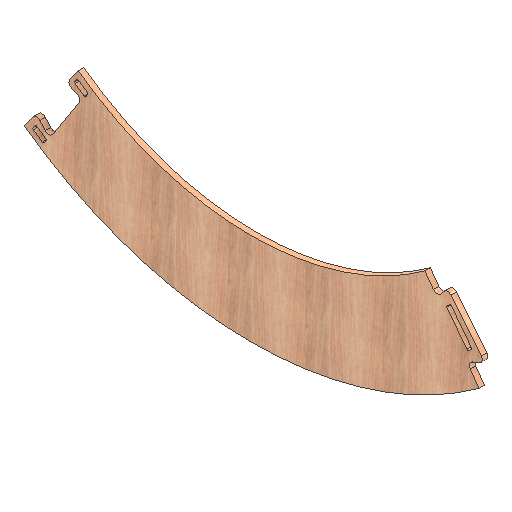
# Autodesk Inventor part: Platform D3
Saved by Autodesk Inventor 2021 (Build 250183000, 183)
## iProperties
Created: 2020-05-09
Part Number: Platform D3
Material: Wood (Birch)
Document SubType Name: Modeling
Designer: Dan Wikman
Density: 0.55 g/cm^3
Appearance: Birch - Natural Polished
Mass: 4202.36 g
Surface Area: 9235.8 cm^2
Volume: 7640.65 cm^3
Autodesk Inventor part; units mm, degrees
ref_plane "YZ Plane" through (0, 0, 0) normal (1, 0, 0) x (0, 1, 0)
ref_plane "XZ Plane" through (0, 0, 0) normal (0, 1, 0) x (-1, 0, 0)
ref_plane "XY Plane" through (0, 0, 0) normal (0, 0, 1) x (1, 0, 0)
sketch "CONTOURS" plane through (0, 0, 0) normal (0, 0, 1) x (1, 0, 0)
  line L0 (1512.926, 262.3244) -> (1483.7011, 302.5491)
  arc A0 (1490.3116, 325.9808) -> (1483.7011, 302.5491) centre (1496.2408, 311.6597) ccw
  line L1 (1490.3116, 325.9808) -> (1515.055, 336.2252)
  arc A1 (1515.055, 336.2252) -> (1520.7765, 358.748) centre (1509.5083, 349.6224) ccw
  line L2 (1520.7765, 358.748) -> (1420.6454, 482.3882)
  arc A2 (1420.6454, 482.3882) -> (1397.875, 482.0914) centre (1409.3772, 473.2625) ccw
  line L3 (1397.875, 482.0914) -> (1387.5892, 468.6913)
  arc A3 (1362.754, 469.0184) -> (1387.5892, 468.6913) centre (1375.2938, 478.1291) ccw
  line L4 (1362.754, 469.0184) -> (1334.3843, 508.066)
  arc A4 (193.4245, 508.066) -> (1334.3843, 508.066) centre (763.9044, 1294.3771) ccw
  line L5 (193.4245, 508.066) -> (165.0547, 469.0184)
  arc A5 (165.0547, 469.0184) -> (171.943, 446.828) centre (176.7854, 460.4955) ccw
  line L6 (171.943, 446.828) -> (187.8658, 441.1866)
  arc A6 (195.6892, 418.1351) -> (187.8658, 441.1866) centre (182.6894, 426.5765) ccw
  line L7 (195.6892, 418.1351) -> (109.0426, 284.6979)
  arc A7 (84.2549, 283.0747) -> (109.0426, 284.6979) centre (96.0429, 293.1392) ccw
  line L8 (84.2549, 283.0747) -> (66.8658, 303.4414)
  arc A8 (66.8658, 303.4414) -> (44.1076, 302.5491) centre (55.8384, 294.0262) ccw
  line L9 (44.1076, 302.5491) -> (14.8827, 262.3244)
  arc A9 (14.8827, 262.3244) -> (1512.926, 262.3244) centre (763.9044, 1294.1149) ccw
  constraints: 20 end point, 20 point on circle, 10 centre point
sketch "HOLES" plane through (0, 0, 0) normal (0, 0, 1) x (1, 0, 0)
  line L0 (224.6944, 455.9957) -> (218.4625, 446.9313)
  arc A0 (212.9002, 445.9014) -> (218.4625, 446.9313) centre (215.1664, 449.1975) ccw
  line L1 (212.9002, 445.9014) -> (183.2349, 466.2968)
  arc A1 (182.205, 471.8591) -> (183.2349, 466.2968) centre (185.5011, 469.5929) ccw
  line L2 (182.205, 471.8591) -> (188.4369, 480.9234)
  arc A2 (193.9992, 481.9534) -> (188.4369, 480.9234) centre (191.733, 478.6573) ccw
  line L3 (193.9992, 481.9534) -> (223.6644, 461.558)
  arc A3 (224.6944, 455.9957) -> (223.6644, 461.558) centre (221.3983, 458.2619) ccw
  line L4 (87.0245, 255.754) -> (80.7926, 246.6896)
  arc A4 (75.2303, 245.6596) -> (80.7926, 246.6896) centre (77.4965, 248.9557) ccw
  line L5 (75.2303, 245.6596) -> (45.5651, 266.055)
  arc A5 (44.5351, 271.6173) -> (45.5651, 266.055) centre (47.8312, 269.3511) ccw
  line L6 (44.5351, 271.6173) -> (50.767, 280.6817)
  arc A6 (56.3293, 281.7117) -> (50.767, 280.6817) centre (54.0631, 278.4155) ccw
  line L7 (56.3293, 281.7117) -> (85.9946, 261.3163)
  arc A7 (87.0245, 255.754) -> (85.9946, 261.3163) centre (83.7284, 258.0201) ccw
  line L8 (1487.4439, 359.9016) -> (1478.716, 353.2066)
  arc A8 (1473.1076, 353.9459) -> (1478.716, 353.2066) centre (1476.2814, 356.3804) ccw
  line L9 (1473.1076, 353.9459) -> (1406.7666, 440.4321)
  arc A9 (1407.5058, 446.0405) -> (1406.7666, 440.4321) centre (1409.9404, 442.8667) ccw
  line L10 (1407.5058, 446.0405) -> (1416.2338, 452.7354)
  arc A10 (1421.8421, 451.9962) -> (1416.2338, 452.7354) centre (1418.6683, 449.5616) ccw
  line L11 (1421.8421, 451.9962) -> (1488.1832, 365.51)
  arc A11 (1487.4439, 359.9016) -> (1488.1832, 365.51) centre (1485.0094, 363.0754) ccw
  constraints: 24 end point, 24 point on circle, 12 centre point
sketch "LETTERS" plane through (0, 0, 0) normal (0, 0, 1) x (1, 0, 0)
  line L0 (221.0345, 299.5651) -> (214.0787, 303.3807)
  line L1 (214.0787, 303.3807) -> (223.8436, 320.6336)
  line L2 (223.8436, 320.6336) -> (229.7881, 317.2691)
  line L3 (232.463, 314.1509) -> (232.5322, 313.9591)
  line L4 (232.5322, 313.9591) -> (232.5968, 313.7631)
  line L5 (232.5968, 313.7631) -> (232.6568, 313.5633)
  line L6 (232.6568, 313.5633) -> (232.7121, 313.3597)
  line L7 (232.7121, 313.3597) -> (232.7625, 313.1525)
  line L8 (232.7625, 313.1525) -> (232.8082, 312.942)
  line L9 (232.8082, 312.942) -> (232.8489, 312.7282)
  line L10 (232.8489, 312.7282) -> (232.8846, 312.5116)
  line L11 (232.8846, 312.5116) -> (232.9153, 312.2921)
  line L12 (232.9153, 312.2921) -> (232.941, 312.0702)
  line L13 (232.941, 312.0702) -> (232.9616, 311.8459)
  line L14 (232.9616, 311.8459) -> (232.9772, 311.6196)
  line L15 (232.9772, 311.6196) -> (232.9877, 311.3915)
  line L16 (232.9877, 311.3915) -> (232.9931, 311.1618)
  line L17 (232.9931, 311.1618) -> (232.9936, 310.9307)
  line L18 (232.9936, 310.9307) -> (232.989, 310.6985)
  line L19 (232.989, 310.6985) -> (232.9795, 310.4654)
  line L20 (232.9795, 310.4654) -> (232.9651, 310.2317)
  line L21 (232.9651, 310.2317) -> (232.9458, 309.9975)
  line L22 (232.9458, 309.9975) -> (232.9218, 309.7632)
  line L23 (232.9218, 309.7632) -> (232.8931, 309.529)
  line L24 (232.8931, 309.529) -> (232.8598, 309.295)
  line L25 (232.8598, 309.295) -> (232.8219, 309.0616)
  line L26 (232.8219, 309.0616) -> (232.7797, 308.8289)
  line L27 (232.7797, 308.8289) -> (232.7331, 308.5971)
  line L28 (232.7331, 308.5971) -> (232.6823, 308.3664)
  line L29 (232.6823, 308.3664) -> (232.6274, 308.1371)
  line L30 (232.6274, 308.1371) -> (232.5686, 307.9094)
  line L31 (232.5686, 307.9094) -> (232.4396, 307.4592)
  line L32 (232.4396, 307.4592) -> (232.2964, 307.0174)
  line L33 (232.2964, 307.0174) -> (232.14, 306.585)
  line L34 (232.14, 306.585) -> (231.9716, 306.1633)
  line L35 (231.9716, 306.1633) -> (231.7923, 305.7532)
  line L36 (231.6033, 305.3555) -> (231.402, 304.9639)
  line L37 (231.402, 304.9639) -> (231.185, 304.5725)
  line L38 (231.185, 304.5725) -> (230.9521, 304.1826)
  line L39 (230.9521, 304.1826) -> (230.7035, 303.7959)
  line L40 (230.7035, 303.7959) -> (230.4394, 303.4138)
  line L41 (230.4394, 303.4138) -> (230.16, 303.038)
  line L42 (230.16, 303.038) -> (230.0147, 302.853)
  line L43 (230.0147, 302.853) -> (229.8658, 302.6702)
  line L44 (229.8658, 302.6702) -> (229.7134, 302.4898)
  line L45 (229.7134, 302.4898) -> (229.5575, 302.3121)
  line L46 (229.5575, 302.3121) -> (229.3982, 302.1372)
  line L47 (229.3982, 302.1372) -> (229.2357, 301.9654)
  line L48 (229.2357, 301.9654) -> (229.07, 301.7969)
  line L49 (229.07, 301.7969) -> (228.9013, 301.6319)
  line L50 (228.9013, 301.6319) -> (228.7297, 301.4705)
  line L51 (228.7297, 301.4705) -> (228.5554, 301.3131)
  line L52 (228.5554, 301.3131) -> (228.3784, 301.1597)
  line L53 (228.3784, 301.1597) -> (228.1989, 301.0107)
  line L54 (228.1989, 301.0107) -> (228.0172, 300.8661)
  line L55 (228.0172, 300.8661) -> (227.8333, 300.7261)
  line L56 (227.8333, 300.7261) -> (227.6474, 300.591)
  line L57 (227.6474, 300.591) -> (227.4598, 300.4608)
  line L58 (227.4598, 300.4608) -> (227.2705, 300.3358)
  line L59 (227.2705, 300.3358) -> (227.0798, 300.2161)
  line L60 (227.0798, 300.2161) -> (226.8878, 300.1017)
  line L61 (226.8878, 300.1017) -> (226.6948, 299.9929)
  line L62 (229.9244, 317.199) -> (230.0598, 317.1238)
  line L63 (230.0598, 317.1238) -> (230.1939, 317.0436)
  line L64 (230.1939, 317.0436) -> (230.3268, 316.9582)
  line L65 (230.3268, 316.9582) -> (230.4581, 316.8676)
  line L66 (230.4581, 316.8676) -> (230.5878, 316.7718)
  line L67 (230.5878, 316.7718) -> (230.7158, 316.6707)
  line L68 (231.7923, 305.7532) -> (231.6033, 305.3555)
  line L69 (230.7158, 316.6707) -> (230.8417, 316.5642)
  line L70 (230.8417, 316.5642) -> (230.9656, 316.4525)
  line L71 (230.9656, 316.4525) -> (231.0872, 316.3353)
  line L72 (231.0872, 316.3353) -> (231.2064, 316.2128)
  line L73 (231.2064, 316.2128) -> (231.3229, 316.085)
  line L74 (221.173, 299.4993) -> (221.0345, 299.5651)
  line L75 (231.3229, 316.085) -> (231.4367, 315.9518)
  line L76 (231.4367, 315.9518) -> (231.5476, 315.8134)
  line L77 (231.5476, 315.8134) -> (231.6554, 315.6696)
  line L78 (231.6554, 315.6696) -> (231.76, 315.5207)
  line L79 (229.7881, 317.2691) -> (229.9244, 317.199)
  line L80 (231.76, 315.5207) -> (231.8612, 315.3665)
  line L81 (231.8612, 315.3665) -> (231.9589, 315.2073)
  line L82 (231.9589, 315.2073) -> (232.0529, 315.0431)
  line L83 (232.0529, 315.0431) -> (232.1431, 314.874)
  line L84 (232.1431, 314.874) -> (232.2293, 314.7001)
  line L85 (232.2293, 314.7001) -> (232.3115, 314.5216)
  line L86 (232.3115, 314.5216) -> (232.3894, 314.3384)
  line L87 (232.3894, 314.3384) -> (232.463, 314.1509)
  line L88 (221.3149, 299.4374) -> (221.173, 299.4993)
  line L89 (221.4601, 299.3795) -> (221.3149, 299.4374)
  line L90 (221.6085, 299.3258) -> (221.4601, 299.3795)
  line L91 (221.7603, 299.2764) -> (221.6085, 299.3258)
  line L92 (221.9152, 299.2315) -> (221.7603, 299.2764)
  line L93 (222.0732, 299.1913) -> (221.9152, 299.2315)
  line L94 (222.2342, 299.1558) -> (222.0732, 299.1913)
  line L95 (222.3983, 299.1252) -> (222.2342, 299.1558)
  line L96 (222.5652, 299.0997) -> (222.3983, 299.1252)
  line L97 (222.7348, 299.0794) -> (222.5652, 299.0997)
  line L98 (222.9072, 299.0644) -> (222.7348, 299.0794)
  line L99 (223.0821, 299.0548) -> (222.9072, 299.0644)
  line L100 (223.2595, 299.0507) -> (223.0821, 299.0548)
  line L101 (223.4391, 299.0523) -> (223.2595, 299.0507)
  line L102 (223.621, 299.0597) -> (223.4391, 299.0523)
  line L103 (223.8049, 299.0728) -> (223.621, 299.0597)
  line L104 (223.9907, 299.0918) -> (223.8049, 299.0728)
  line L105 (224.1783, 299.1168) -> (223.9907, 299.0918)
  line L106 (224.3674, 299.1478) -> (224.1783, 299.1168)
  line L107 (224.5579, 299.1849) -> (224.3674, 299.1478)
  line L108 (224.7497, 299.228) -> (224.5579, 299.1849)
  line L109 (224.9425, 299.2773) -> (224.7497, 299.228)
  line L110 (225.1362, 299.3327) -> (224.9425, 299.2773)
  line L111 (225.3306, 299.3942) -> (225.1362, 299.3327)
  line L112 (225.5256, 299.4618) -> (225.3306, 299.3942)
  line L113 (225.7208, 299.5354) -> (225.5256, 299.4618)
  line L114 (225.9161, 299.6151) -> (225.7208, 299.5354)
  line L115 (226.1114, 299.7008) -> (225.9161, 299.6151)
  line L116 (226.3064, 299.7923) -> (226.1114, 299.7008)
  line L117 (226.5009, 299.8898) -> (226.3064, 299.7923)
  line L118 (226.6948, 299.9929) -> (226.5009, 299.8898)
  constraints: 238 end point
extrude "Extrusion1" add sketch "CONTOURS" along normal blind 18
extrude "Extrusion2" cut sketch "HOLES" along normal blind 18
body "Solid1"
